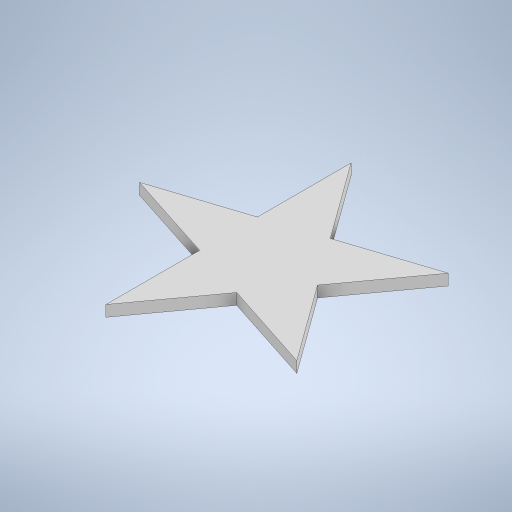
# Autodesk Inventor part: Estrella
Saved by Autodesk Inventor 2023 (Build 270158000, 158)
## iProperties
Created: 2024-12-19
Part Number: Estrella
Material: Genérico
Document SubType Name: Modeling
Designer: Osqui Alvareto
Density: 1 g/cm^3
Appearance: Valor por defecto
Author: Osqui Alvareto
Autodesk Inventor part; units mm, degrees
ref_plane "YZ Plane" through (0, 0, 0) normal (1, 0, 0) x (0, 1, 0)
ref_plane "XZ Plane" through (0, 0, 0) normal (0, 1, 0) x (-1, 0, 0)
ref_plane "XY Plane" through (0, 0, 0) normal (0, 0, 1) x (1, 0, 0)
sketch "Boceto1" plane through (0, 0, 0) normal (0, 1, 0) x (-1, 0, 0)
  circle A0 centre (0, 0) radius 35
  line L0 (35, 0) -> (10.8156, -33.287)
  line L1 (10.8156, -33.287) -> (-28.3156, -20.5725)
  line L2 (-28.3156, -20.5725) -> (-28.3156, 20.5725)
  line L3 (-28.3156, 20.5725) -> (10.8156, 33.287)
  line L4 (10.8156, 33.287) -> (35, 0)
  line L5 (35, 0) -> (-28.3156, -20.5725)
  line L6 (10.8156, 33.287) -> (10.8156, -33.287)
  line L7 (10.8156, -33.287) -> (-28.3156, 20.5725)
  line L8 (35, 0) -> (-28.3156, 20.5725)
  line L9 (-28.3156, -20.5725) -> (10.8156, 33.287)
  point P0 (10.8156, 7.858)
  point P1 (-4.1312, 12.7145)
  point P2 (-13.3688, 0)
  point P3 (-4.1312, -12.7145)
  point P4 (10.8156, -7.858)
  dimension "d0" = 70
  constraints: 20 end point, 3 point on circle, 2 coincident, 1 centre point, 1 point on line, 1 vertical, 11 other
  measures "d0" diameter of A0
extrude "Extrusión1" add sketch "Boceto1" along normal blind 3 contours L5 L6 L8 | L6 L8 L9 | L7 L5 L6 | L5 L7 L9 L8 L6 | L8 L9 L7 | L9 L7 L5
